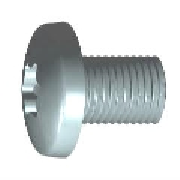
# Autodesk Inventor part: Flachkopfschraube mit Innenrund ISO 14583 - M2,5 x 8 - A2-70
Saved by Autodesk Inventor 2023 (Build 270158000, 158)
## iProperties
Created: 2022-02-04
Part Number: Flachkopfschraube mit Innenrund ISO 14583 - M2,5 x 8 - A2-70
Material: Edelstahl
Description: Flachkopfschrauben mit Innenrund ISO 14583
Document SubType Name: Modeling
Standard: 14583
Designer: jan
Standards Organization: ISO
Language: de-DE
Size Designation: M2,5x8-A2-70
Categories: <MemberInstance><Categories><Category DisplayName="Verbindungselemente" InternalName="e4da775c-781d-43d5-af7c-5136215cf5a6" Mnemonic="FSTN"><Category DisplayName="Schrauben" InternalName="536e6df0-f778-49ac-b2f2-25c71d2aa0b2" Mnemonic="SCRW"><CategoryParameter DisplayName="Bezeichnung des Nenndurchmessers" InternalName="03caf894-eafd-4c09-a035-916ac084b87b" Mnemonic="nomdiadesig"/><CategoryParameter DisplayName="Nennlänge" InternalName="238ecbaf-3e6c-45dd-aa95-4068c8e0fd02" Mnemonic="nomlen"/><CategoryParameter DisplayName="Gewindebezeichnung" InternalName="586d5e89-370a-4089-914f-0110033585c7" Mnemonic="thrdesign"/><CategoryParameter DisplayName="Gewindeserienbeschreibung" InternalName="87c5849c-b3a5-4c3e-9c9b-2feecef9be86" Mnemonic="thrserdsgn"/><CategoryParameter DisplayName="Nenndurchmesser" InternalName="8bbe3f8e-44cf-40a9-a251-3a6edc8168d6" Mnemonic="nomdia"/><CategoryParameter DisplayName="Gewindeart" InternalName="b4bbb7bc-d6aa-4c9f-a9a9-4152b9f6fe49" Mnemonic="thrtype"/><CategoryParameter DisplayName="Gewindesteigung" InternalName="bb82302e-82d8-4176-8fc1-c5d7bb17d5ad" Mnemonic="pitch1"/><CategoryParameter DisplayName="Windungen pro Einheit" InternalName="bdc6e7d2-ffd0-4d9c-a173-16b95ebb912d" Mnemonic="thrperunit1"/><CategoryParameter DisplayName="Gewindeklasse" InternalName="ebc0d23b-2cc6-4d2a-b376-d52aae53bab6" Mnemonic="thrclss"/><Category DisplayName="Rundkopf" InternalName="df3578aa-538f-4805-96a8-2439eb0c3cf7" Mnemonic="RNDSCRW"><CategoryParameter DisplayName="Grifflänge" InternalName="2c6ace26-543b-4217-91c4-9cdf8c3ec6f1" Mnemonic="grplen"/><CategoryParameter DisplayName="Kopfhöhe" InternalName="2d152238-84fe-49ae-94c3-3fee884c292b" Mnemonic="headh"/><CategoryParameter DisplayName="Eigenschaftenklasse" InternalName="85496db6-1567-48ed-b0d4-aa1f03366005" Mnemonic="propclss"/><CategoryParameter DisplayName="Gewindelänge" InternalName="a1e5edc5-4ca7-4847-8786-65b14d35af16" Mnemonic="thrlen"/><CategoryParameter DisplayName="Schaftdurchmesser" InternalName="c22f1a48-b8d5-43ef-ac5e-546ba91c0bd6" Mnemonic="grpdia"/><CategoryParameter DisplayName="Kopfdurchmesser" InternalName="e71ee7a1-06fd-425c-ba3b-09769885677c" Mnemonic="headdia"/></Category></Category></Category><Category DisplayName="Datentyp" InternalName="23b78d0f-2648-40c6-8793-ca6db495c9e8" Mnemonic="DATATYPE"><CategoryParameter DisplayName="Anzeigename" InternalName="05415f3d-3907-474b-a020-eb9d644f4cf3" Mnemonic="DISPLAYNAME"/><CategoryParameter DisplayName="Norm" InternalName="0c0a119c-1e12-4c84-803f-101930972f5e" Mnemonic="STANDARD"/><CategoryParameter DisplayName="Beschreibung" InternalName="13903e3d-64b1-4950-80da-f627842ea37f" Mnemonic="DESCRIPTION"/><CategoryParameter DisplayName="Bezeichnung" InternalName="2675968c-4ce5-49e0-a4f5-552d29089031" Mnemonic="DESIGNATION"/><CategoryParameter DisplayName="Standardzeile" InternalName="2af9ec52-faaa-4026-b378-f9fa4afca842" Mnemonic="DEFAULTROW"/><CategoryParameter DisplayName="Ordnername" InternalName="3f06958e-8713-4116-9be7-ed6184ecc97b" Mnemonic="FOLDERNAME"/><CategoryParameter DisplayName="Revisionsanleitung" InternalName="45a75005-10b1-4dfc-8d6d-dfe629f0b93c" Mnemonic="REVISIONGUID"/><CategoryParameter DisplayName="Dateiname" InternalName="8b46a4cc-9585-4fed-90c3-899f57e09a73" Mnemonic="FILENAME"/><CategoryParameter DisplayName="Normungsorganisation" InternalName="8f5914e1-4693-403f-8ab5-d37768198c9d" Mnemonic="STDSORG"/><CategoryParameter DisplayName="Gruppenversion" InternalName="914462f6-6e19-4b14-ba84-155b9680b1d0" Mnemonic="FAMILYREVISION"/><CategoryParameter DisplayName="Normrevision" InternalName="91d5a463-65c2-4fde-b823-3b7fea5e8e17" Mnemonic="STANDARDREVISION"/><CategoryParameter DisplayName="Variantenrevision" InternalName="a65d44b9-392f-4f4f-857b-e4b3d54996fe" Mnemonic="MEMBERREVISION"/><CategoryParameter DisplayName="ClipFormat" InternalName="bc51e27b-3422-4e78-93ef-cec197ddf230" Mnemonic="CLIPFORMAT"/><CategoryParameter DisplayName="Hersteller" InternalName="cd6c7a72-a28a-4e50-99a9-2c7f4e13e5ad" Mnemonic="MANUFACTURER"/><CategoryParameter DisplayName="InternerName" InternalName="cf1d0246-76d9-4b4a-8305-fa0409afb5c1" Mnemonic="INTERNALNAME"/><CategoryParameter DisplayName="IstMetrisch" InternalName="e2385c5b-1ea4-4823-96a8-8de651266ec3" Mnemonic="ISMETRIC"/><Category DisplayName="Bauteil" InternalName="c0e0b642-3bcb-4cc8-9e80-f96d35c4afa4" Mnemonic="PART"><CategoryParameter DisplayName="Bauteilnummer" InternalName="016b6077-bfbe-49bd-92c9-d8d59c39c941" Mnemonic="PARTNUMBER"/><CategoryParameter DisplayName="Bestandsnummer" InternalName="4dba7c1c-e26c-444e-836c-b08b433409a8" Mnemonic="STOCKNUMBER"/><CategoryParameter DisplayName="Materialschlüssel" InternalName="5c9a8adb-dd2b-4535-b97f-0a94a95fe41f" Mnemonic="MATERIALKEY"/><CategoryParameter DisplayName="Material" InternalName="818a152a-d3c3-49ca-80ee-df7d91421b8e" Mnemonic="MATERIAL"/></Category></Category></Categories><FamilyTemplate Id="ISO14583"><FamilyTemplateParameters><FamilyTemplateParameter ObjectType="kUserParameterObject" ValueType="xs:double" Id="36" ObjectReferenceKey="lg"/><FamilyTemplateParameter ObjectType="kUserParameterObject" ValueType="xs:double" Id="37" ObjectReferenceKey="dk"/><FamilyTemplateParameter ObjectType="kUserParameterObject" ValueType="xs:double" Id="38" ObjectReferenceKey="k"/><FamilyTemplateParameter ObjectType="kUserParameterObject" ValueType="xs:double" Id="39" ObjectReferenceKey="d"/><FamilyTemplateParameter ObjectType="kUserParameterObject" ValueType="xs:double" Id="40" ObjectReferenceKey="l_"/><FamilyTemplateParameter ObjectType="kUserParameterObject" ValueType="xs:double" Id="41" ObjectReferenceKey="b"/><FamilyTemplateParameter ObjectType="kUserParameterObject" ValueType="xs:double" Id="63" ObjectReferenceKey="A_"/><FamilyTemplateParameter ObjectType="kUserParameterObject" ValueType="xs:double" Id="65" ObjectReferenceKey="rf"/><FamilyTemplateParameter ObjectType="kUserParameterObject" ValueType="xs:double" Id="66" ObjectReferenceKey="r"/><FamilyTemplateParameter ObjectType="kUserParameterObject" ValueType="xs:double" Id="67" ObjectReferenceKey="t"/><FamilyTemplateParameter ObjectType="kUserParameterObject" ValueType="xs:double" Id="68" ObjectReferenceKey="x"/><FamilyTemplateParameter ObjectType="kUserParameterObject" ValueType="xs:double" Id="92" ObjectReferenceKey="p"/><FamilyTemplateParameter ObjectType="kThreadFeatureObject" ValueType="xs:string" Id="89" ObjectReferenceKey="1002000010000000767c0100000000008000000000000000" SubObjectId="ThreadInfo"><FamilyTemplateParameter ObjectType="" ValueType="xs:string" Id="90" SubObjectId="ThreadClass"/><FamilyTemplateParameter ObjectType="" ValueType="xs:string" Id="91" SubObjectId="ThreadDesignation"/><FamilyTemplateParameter ObjectType="" ValueType="xs:string" Id="93" SubObjectId="ThreadType"/></FamilyTemplateParameter><FamilyTemplateParameter ObjectType="kPartComponentDefinitionObject" ValueType="xs:string" Id="104" SubObjectId="Material"/><FamilyTemplateParameter ObjectType="kPropertyObject" ValueType="xs:string" Id="113" ObjectReferenceKey="{32853F0F-3444-11d1-9E93-0060B03C1CA6}" SubObjectId="5"/><FamilyTemplateParameter ObjectType="kPropertyObject" ValueType="xs:string" Id="114" ObjectReferenceKey="{32853F0F-3444-11d1-9E93-0060B03C1CA6}" SubObjectId="52"/></FamilyTemplateParameters></FamilyTemplate><CategoryParameterMap><ParamToTemplateMap><ParamToTemplate CategoryParameter="//CategoryParameter[@InternalName='cf1d0246-76d9-4b4a-8305-fa0409afb5c1']" ConstantValue="35dccc23-f369-4e39-b76e-30ef466fa2fb"/><ParamToTemplate CategoryParameter="//CategoryParameter[@InternalName='45a75005-10b1-4dfc-8d6d-dfe629f0b93c']" ConstantValue="eaa99e2c-6c48-4f01-a64d-ac7d293135d6"/><ParamToTemplate CategoryParameter="//CategoryParameter[@InternalName='3f06958e-8713-4116-9be7-ed6184ecc97b']" ConstantValue="ISO 14583"/><ParamToTemplate CategoryParameter="//CategoryParameter[@InternalName='8f5914e1-4693-403f-8ab5-d37768198c9d']" ConstantValue="ISO"/><ParamToTemplate CategoryParameter="//CategoryParameter[@InternalName='0c0a119c-1e12-4c84-803f-101930972f5e']" ConstantValue="14583"/><ParamToTemplate CategoryParameter="//CategoryParameter[@InternalName='91d5a463-65c2-4fde-b823-3b7fea5e8e17']" TemplateParameter="100"/><ParamToTemplate CategoryParameter="//CategoryParameter[@InternalName='cd6c7a72-a28a-4e50-99a9-2c7f4e13e5ad']" TemplateParameter="101"/><ParamToTemplate CategoryParameter="//CategoryParameter[@InternalName='13903e3d-64b1-4950-80da-f627842ea37f']" ConstantValue="Hexalobular socket pan head screws ISO 14583"/><ParamToTemplate CategoryParameter="//CategoryParameter[@InternalName='05415f3d-3907-474b-a020-eb9d644f4cf3']" ConstantValue="Screw ISO 14583:2011(E)"/><ParamToTemplate CategoryParameter="//CategoryParameter[@InternalName='914462f6-6e19-4b14-ba84-155b9680b1d0']" ConstantValue="11"/><ParamToTemplate CategoryParameter="//CategoryParameter[@InternalName='bc51e27b-3422-4e78-93ef-cec197ddf230']" ConstantValue="CF_INVENTOR.STDPARTS"/><ParamToTemplate CategoryParameter="//CategoryParameter[@InternalName='e2385c5b-1ea4-4823-96a8-8de651266ec3']" ConstantValue="true"/><ParamToTemplate CategoryParameter="//CategoryParameter[@InternalName='2af9ec52-faaa-4026-b378-f9fa4afca842']" ConstantValue="1"/><ParamToTemplate CategoryParameter="//CategoryParameter[@InternalName='8b46a4cc-9585-4fed-90c3-899f57e09a73']" ConstantValue="ISO 14583 - M2,5x8-A2-70"/><ParamToTemplate CategoryParameter="//CategoryParameter[@InternalName='a65d44b9-392f-4f4f-857b-e4b3d54996fe']" ConstantValue="0EF35504-9F20-4A99-A62F-294D07470BA3"/><ParamToTemplate CategoryParameter="//CategoryParameter[@InternalName='a65d44b9-392f-4f4f-857b-e4b3d54996fe']" ConstantValue="0EF35504-9F20-4A99-A62F-294D07470BA3"/><ParamToTemplate CategoryParameter="//CategoryParameter[@InternalName='2675968c-4ce5-49e0-a4f5-552d29089031']" TemplateParameter="114"/><ParamToTemplate CategoryParameter="//CategoryParameter[@InternalName='a1e5edc5-4ca7-4847-8786-65b14d35af16']" TemplateParameter="41"/><ParamToTemplate CategoryParameter="//CategoryParameter[@InternalName='e71ee7a1-06fd-425c-ba3b-09769885677c']" TemplateParameter="37"/><ParamToTemplate CategoryParameter="//CategoryParameter[@InternalName='2d152238-84fe-49ae-94c3-3fee884c292b']" TemplateParameter="38"/><ParamToTemplate CategoryParameter="//CategoryParameter[@InternalName='2c6ace26-543b-4217-91c4-9cdf8c3ec6f1']" TemplateParameter="36"/><ParamToTemplate CategoryParameter="//CategoryParameter[@InternalName='818a152a-d3c3-49ca-80ee-df7d91421b8e']" TemplateParameter="104"/><ParamToTemplate CategoryParameter="//CategoryParameter[@InternalName='238ecbaf-3e6c-45dd-aa95-4068c8e0fd02']" TemplateParameter="40"/><ParamToTemplate CategoryParameter="//CategoryParameter[@InternalName='8bbe3f8e-44cf-40a9-a251-3a6edc8168d6']" TemplateParameter="39"/><ParamToTemplate CategoryParameter="//CategoryParameter[@InternalName='016b6077-bfbe-49bd-92c9-d8d59c39c941']" TemplateParameter="113"/><ParamToTemplate CategoryParameter="//CategoryParameter[@InternalName='bb82302e-82d8-4176-8fc1-c5d7bb17d5ad']" TemplateParameter="92"/><ParamToTemplate CategoryParameter="//CategoryParameter[@InternalName='ebc0d23b-2cc6-4d2a-b376-d52aae53bab6']" TemplateParameter="90"/><ParamToTemplate CategoryParameter="//CategoryParameter[@InternalName='586d5e89-370a-4089-914f-0110033585c7']" TemplateParameter="91"/><ParamToTemplate CategoryParameter="//CategoryParameter[@InternalName='b4bbb7bc-d6aa-4c9f-a9a9-4152b9f6fe49']" TemplateParameter="93"/></ParamToTemplateMap></CategoryParameterMap></MemberInstance>
Mass: 0.565862 g
Surface Area: 1.30141 cm^2
Volume: 0.0707327 cm^3
Density: 8 g/cm^3
Appearance: Plate
IsCustomPart: 0
Author: jan
Autodesk Inventor part; units mm, degrees
ref_plane "YZ Plane" through (0, 0, 0) normal (1, 0, 0) x (0, 1, 0)
ref_plane "XZ Plane" through (0, 0, 0) normal (0, 1, 0) x (-1, 0, 0)
ref_plane "XY Plane" through (0, 0, 0) normal (0, 0, 1) x (1, 0, 0)
sketch "Sketch4" plane through (0, 0, 0) normal (0, 0, 1) x (1, 0, 0)
  line L0 (-2.1, 0) -> (8, 0)
  line L1 (0, 0) -> (-2.1, 0)
  line L2 (0, 2.5) -> (0, 1.625)
  line L3 (0.4, 1.225) -> (0.4, 1.225)
  line L4 (0.4, 1.225) -> (0.8, 1.25)
  arc A0 (0, 1.625) -> (0.4, 1.225) centre (0.4, 1.625) ccw
  line L5 (-2.1, 0) -> (-2.1, 1.25)
  line L6 (0, 2.5) -> (-1.1375, 2.5)
  arc A1 (-1.1375, 2.5) -> (-2.1, 1.25) centre (1.4883, -0.5175) ccw
  line L7 (0.8, 1.25) -> (8, 1.25)
  line L8 (8, 1.25) -> (8, 0)
  point P0 (0, 1.225)
  dimension "d71" = 0.4
  dimension "d72" = 8
  dimension "d74" = 0.4
  dimension "d75" = 2.45
  dimension "d78" = 2.5
  dimension "d82" = 4
  dimension "d83" = 2.1
  dimension "d84" = 5
  dimension "d104" = 7.2
  dimension "d105" = 2.5
  constraints: 18 end point, 5 point on line, 4 horizontal, 4 point on circle, 2 centre point, 2 tangent, 1 perpendicular, 1 vertical
  measures "d71" radius of A0
  measures "d72" distance of L0.end L1.start
  measures "d74" horizontal distance of L3.end L4.end
  measures "d75" diameter of L3 L0
  measures "d78" diameter of L5.end L0
  measures "d82" radius of A1
  measures "d83" distance between parallel lines of L2 L5
  measures "d84" diameter of L6 L0
  measures "d104" distance of L4.end L7.end
  measures "d105" diameter of L7.end L0
revolve "Revolution7" add sketch "Sketch4" angle 360 about axis through (-2.1, 0, 0) along (1, 0, 0)
sketch "Sketch5" plane through (-2.1, 0, 0) normal (-1, 0, 0) x (0, 0, 1)
  circle A0 centre (0, 0) radius 1.2 construction
  circle A1 centre (0, 0) radius 0.84 construction
  line L0 (0, 0) -> (-0.7275, 0.42)
  line L1 (0, 0) -> (-0.7275, -0.42)
  line L2 (-1.8008, 0) -> (1.7887, 0)
  line L3 (-1.2, 0) -> (-0.7275, -0.42)
  line L4 (-1.2, 0) -> (-0.7275, 0.42)
  dimension "d88" = 2.4
  dimension "d89" = 1.68
  dimension "d90" = 30
  dimension "d91" = 30
  constraints: 10 end point, 3 coincident, 2 point on circle, 2 point on line, 1 centre point, 1 horizontal, 1 horizontal alignment, 2 other
  measures "d89" diameter of A1
  measures "d90" angle of L2 L0
  measures "d91" angle of L2 L1
extrude "Extrusion1" cut sketch "Sketch5" against normal blind 1.04
pattern_circular "Circular Pattern1" count 6 over 360 about axis through (-10, 0, 0) along (1, 0, 0) of "Extrusion1"
fillet "Fillet1" radius 0.24 12 edges at (-1.58, -1.0392, -0.6) (-1.58, -0.42, -0.7275) (-1.58, -0.84, 0) (-1.58, -1.0392, 0.6) (-1.58, -0.42, 0.7275) (-1.58, 0, 1.2) (-1.58, 0.84, 0) (-1.58, 1.0392, 0.6) (-1.58, 0.42, 0.7275) (-1.58, 0.42, -0.7275) (-1.58, 0, -1.2) (-1.58, 1.0392, -0.6)
thread "Thread7" size "M2.5x0.45" class "6g" standard "ISO Metric profile" length 7.2
body "Solid7"
